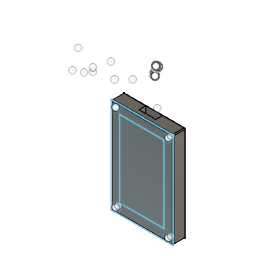
macropad-design 3.0 (Autodesk Fusion 360 design; units mm, degrees)
part number: 2025-12-03-17-34-09-700
part number: 2026-05-21-03-28-54-100
Autodesk Fusion 360 part; units mm, degrees
sketch "Sketch1" plane through (0, 0, 0) normal (0, 1, 0) x (1, 0, 0)
  line L0 (-41.1708, 57.3999) -> (7.4423, 57.3999)
  line L1 (7.4423, 57.3999) -> (7.4423, 141.552)
  line L2 (7.4423, 141.552) -> (-41.1708, 141.552)
  line L3 (-41.1708, 141.552) -> (-41.1708, 57.3999)
  line L4 (-50.6708, 47.8999) -> (17.375, 47.8999)
  line L5 (17.375, 47.8999) -> (17.375, 152.9579)
  line L6 (17.375, 152.9579) -> (-50.6708, 152.9579)
  line L7 (-50.6708, 152.9579) -> (-50.6708, 47.8999)
  circle A0 centre (-45.6708, 147.9579) radius 1.7
  circle A1 centre (-45.6708, 52.8999) radius 1.7
  circle A2 centre (12.375, 52.8999) radius 1.7
  circle A3 centre (12.375, 147.9579) radius 1.7
  circle A4 centre (-45.6708, 52.8999) radius 3
  circle A5 centre (12.375, 52.8999) radius 3
  circle A6 centre (12.375, 147.9579) radius 3
  circle A7 centre (-45.6708, 147.9579) radius 3
  dimension "d1" = 105.058
  dimension "d2" = 68.0458
  dimension "d3" = 48.6131
  dimension "d4" = 84.1522
  dimension "d5" = 9.5
  dimension "d6" = 9.5
  dimension "d7" = 3.4
  dimension "d8" = 5
  dimension "d9" = 5
  dimension "d10" = 3.4
  dimension "d11" = 5
  dimension "d12" = 5
  dimension "d13" = 3.4
  dimension "d14" = 5
  dimension "d15" = 5
  dimension "d16" = 3.4
  dimension "d17" = 5
  dimension "d18" = 5
  dimension "d19" = 6
  dimension "d20" = 6
  dimension "d21" = 6
  dimension "d22" = 6
  constraint horizontal L0
  constraint vertical L1
  constraint horizontal L2
  constraint vertical L3
  constraint horizontal L4
  constraint vertical L5
  constraint horizontal L6
  constraint vertical L7
  constraint concentric A1 A4
  constraint concentric A2 A5
  constraint concentric A3 A6
  constraint concentric A0 A7
  measures "d1" distance of L4.end L5.end
  measures "d2" distance of L4.start L4.end
  measures "d3" distance of L0.start L0.end
  measures "d4" distance of L0.start L2.end
  measures "d5" distance of L3 L7
  measures "d6" distance of L0 L4
  measures "d7" diameter of A0
  measures "d8" distance of L7 A0.centre
  measures "d9" distance of L6 A0.centre
  measures "d10" diameter of A1
  measures "d11" distance of L7 A1.centre
  measures "d12" distance of L4 A1.centre
  measures "d13" diameter of A2
  measures "d14" distance of L5 A2.centre
  measures "d15" distance of L4 A2.centre
  measures "d16" diameter of A3
  measures "d17" distance of L6 A3.centre
  measures "d18" distance of L5 A3.centre
  measures "d19" diameter of A4
  measures "d20" diameter of A5
  measures "d21" diameter of A6
  measures "d22" diameter of A7
extrude "Extrude1" add sketch "Sketch1" along normal blind 9.9 from surface at 3.1 contours A4 | A5 | A6 | A7 makes body 1 at (-48.667, 9.7, -52.7503) makes body 2 at (-42.9063, 9.7, -149.1232) makes body 3 at (15.3713, 9.7, -52.7503) makes body 4 at (9.6106, 9.7, -149.1232)
extrude "Extrude2" add sketch "Sketch1" along normal blind 13 contours L4 L5 L6 L7 bodies 1 2 3 4
extrude "Extrude3" add sketch "Sketch1" along normal blind 3 contours L0 L1 L2 L3 bodies 1
sketch "Sketch2" plane through (0, 13, 0) normal (0, 1, 0) x (-1, 0, 0)
  circle A0 centre (45.6708, -52.8999) radius 1.7
  circle A1 centre (-12.375, -147.9579) radius 1.7
  line L0 (41.1708, -57.3999) -> (41.1708, -141.552)
  line L1 (41.1708, -141.552) -> (-7.4423, -141.552)
  line L2 (-7.4423, -141.552) -> (-7.4423, -57.3999)
  line L3 (-7.4423, -57.3999) -> (41.1708, -57.3999)
  line L4 (50.6708, -152.9579) -> (50.6708, -47.8999)
  line L5 (50.6708, -47.8999) -> (-17.375, -47.8999)
  line L6 (-17.375, -47.8999) -> (-17.375, -152.9579)
  line L7 (-17.375, -152.9579) -> (50.6708, -152.9579)
  circle A2 centre (45.6708, -147.9579) radius 1.7
  circle A3 centre (-12.375, -52.8999) radius 1.7
  line L8 (7.175, -47.8999) -> (25.675, -47.8999)
  line L9 (25.675, -47.8999) -> (25.675, -57.3999)
  line L10 (25.675, -57.3999) -> (7.175, -57.3999)
  line L11 (7.175, -57.3999) -> (7.175, -47.8999)
  line L12 (-17.375, -47.8999) -> (-17.375, -152.9579)
  line L13 (-17.375, -152.9579) -> (50.6708, -152.9579)
  line L14 (50.6708, -152.9579) -> (50.6708, -47.8999)
  line L15 (50.6708, -47.8999) -> (-17.375, -47.8999)
  line L16 (-17.375, -47.8999) -> (-17.375, -152.9579)
  point P0 (50.6708, -152.9579)
  point P1 (-17.375, -152.9579)
  point P2 (50.6708, -47.8999)
  point P3 (-17.375, -47.8999)
  dimension "d30" = 18.5
  dimension "d32" = 24.55
  constraint horizontal L8
  constraint vertical L9
  constraint horizontal L10
  constraint vertical L11
  constraint coincident L5 L8.start
  measures "d30" distance of L8.start L8.end
  measures "d32" distance of L11 L12
extrude "Extrude4" cut sketch "Sketch2" against normal blind 7.5 contours L3 L5 L8 L9 L10 L11 L15 bodies 1
sketch "Sketch3" plane through (0, 0, 0) normal (0, 1, 0) x (1, 0, 0)
sketch "Sketch4" plane through (0, 3, 0) normal (0, 1, 0) x (-1, 0, 0)
  line L0 (41.1708, -141.552) -> (41.1708, -57.3999)
  line L1 (41.1708, -57.3999) -> (-7.4423, -57.3999)
  line L2 (-7.4423, -57.3999) -> (-7.4423, -141.552)
  line L3 (-7.4423, -141.552) -> (41.1708, -141.552)
  line L4 (6.8441, -1.7803) -> (6.8447, -1.7809)
  line L5 (6.8447, -1.7809) -> (6.8447, -1.7812)
  line L6 (6.8447, -1.7812) -> (6.8447, -5.0625)
  line L7 (6.8447, -5.0625) -> (6.8447, -5.0629)
  line L8 (6.8447, -5.0629) -> (6.8441, -5.0634)
  line L9 (6.8441, -5.0634) -> (6.8438, -5.0635)
  line L10 (6.8438, -5.0635) -> (4.9688, -5.0635)
  line L11 (4.9688, -5.0635) -> (4.9684, -5.0634)
  line L12 (4.9684, -5.0634) -> (4.9678, -5.0629)
  line L13 (4.9678, -5.0629) -> (4.9678, -5.0625)
  line L14 (4.9678, -5.0625) -> (4.9678, -1.7812)
  line L15 (4.9678, -1.7812) -> (4.9678, -1.7809)
  line L16 (4.9678, -1.7809) -> (4.9684, -1.7803)
  line L17 (4.9684, -1.7803) -> (4.9688, -1.7803)
  line L18 (4.9688, -1.7803) -> (6.8438, -1.7803)
  line L19 (6.8438, -1.7803) -> (6.8441, -1.7803)
  line L20 (4.9697, -1.7822) -> (4.9697, -5.0615)
  line L21 (4.9697, -5.0615) -> (6.8428, -5.0615)
  line L22 (6.8428, -5.0615) -> (6.8428, -1.7822)
  line L23 (6.8428, -1.7822) -> (4.9697, -1.7822)
  circle A0 centre (6.75, -4.9688) radius 0.0433
  circle A1 centre (5.0625, -4.9688) radius 0.0433
  circle A2 centre (6.75, -1.875) radius 0.0433
  circle A3 centre (5.0625, -1.875) radius 0.0433
  circle A4 centre (5.3312, -3.0938) radius 0.0335
  circle A5 centre (5.5312, -3.0938) radius 0.0787
  circle A6 centre (5.7313, -3.0938) radius 0.0335
  circle A7 centre (5.6312, -2.8937) radius 0.0295
  circle A8 centre (5.3812, -2.9937) radius 0.0295
  circle A9 centre (6.0813, -3.0938) radius 0.0335
  circle A10 centre (6.2812, -3.0938) radius 0.0787
  circle A11 centre (6.4813, -3.0938) radius 0.0335
  circle A12 centre (6.3813, -2.8937) radius 0.0295
  circle A13 centre (6.1313, -2.9937) radius 0.0295
  circle A14 centre (5.5858, -1.8956) radius 0.0175
  circle A15 centre (5.5858, -1.9956) radius 0.0175
  circle A16 centre (5.5858, -2.0956) radius 0.0175
  circle A17 centre (5.5858, -2.1956) radius 0.0175
  circle A18 centre (5.5858, -2.2956) radius 0.0175
  circle A19 centre (5.5858, -2.3956) radius 0.0175
  circle A20 centre (5.5858, -2.4956) radius 0.0175
  circle A21 centre (6.1858, -2.4956) radius 0.0175
  circle A22 centre (6.1858, -2.3956) radius 0.0175
  circle A23 centre (6.1858, -2.2956) radius 0.0175
  circle A24 centre (6.1858, -2.1956) radius 0.0175
  circle A25 centre (6.1858, -2.0956) radius 0.0175
  circle A26 centre (6.1858, -1.9956) radius 0.0175
  circle A27 centre (6.1858, -1.8956) radius 0.0175
  circle A28 centre (6.0813, -3.8438) radius 0.0335
  circle A29 centre (6.2812, -3.8438) radius 0.0787
  circle A30 centre (6.4813, -3.8438) radius 0.0335
  circle A31 centre (6.3813, -3.6437) radius 0.0295
  circle A32 centre (6.1313, -3.7438) radius 0.0295
  circle A33 centre (5.3312, -3.8438) radius 0.0335
  circle A34 centre (5.5312, -3.8438) radius 0.0787
  circle A35 centre (5.7313, -3.8438) radius 0.0335
  circle A36 centre (5.6312, -3.6437) radius 0.0295
  circle A37 centre (5.3812, -3.7438) radius 0.0295
  circle A38 centre (5.3312, -4.5938) radius 0.0335
  circle A39 centre (5.5312, -4.5938) radius 0.0787
  circle A40 centre (5.7313, -4.5938) radius 0.0335
  circle A41 centre (5.6312, -4.3937) radius 0.0295
  circle A42 centre (5.3812, -4.4938) radius 0.0295
  circle A43 centre (6.75, -4.9688) radius 0.0433
  circle A44 centre (5.0625, -4.9688) radius 0.0433
  circle A45 centre (6.75, -1.875) radius 0.0433
  circle A46 centre (5.0625, -1.875) radius 0.0433
  circle A47 centre (5.3312, -3.0938) radius 0.0335
  circle A48 centre (5.5312, -3.0938) radius 0.0787
  circle A49 centre (5.7313, -3.0938) radius 0.0335
  circle A50 centre (5.6312, -2.8937) radius 0.0295
  circle A51 centre (5.3812, -2.9937) radius 0.0295
  circle A52 centre (6.0813, -3.0938) radius 0.0335
  circle A53 centre (6.2812, -3.0938) radius 0.0787
  circle A54 centre (6.4813, -3.0938) radius 0.0335
  circle A55 centre (6.3813, -2.8937) radius 0.0295
  circle A56 centre (6.1313, -2.9937) radius 0.0295
  circle A57 centre (5.5858, -1.8956) radius 0.0175
  circle A58 centre (5.5858, -1.9956) radius 0.0175
  circle A59 centre (5.5858, -2.0956) radius 0.0175
  circle A60 centre (5.5858, -2.1956) radius 0.0175
  circle A61 centre (5.5858, -2.2956) radius 0.0175
  circle A62 centre (5.5858, -2.3956) radius 0.0175
  circle A63 centre (5.5858, -2.4956) radius 0.0175
  circle A64 centre (6.1858, -2.4956) radius 0.0175
  circle A65 centre (6.1858, -2.3956) radius 0.0175
  circle A66 centre (6.1858, -2.2956) radius 0.0175
  circle A67 centre (6.1858, -2.1956) radius 0.0175
  circle A68 centre (6.1858, -2.0956) radius 0.0175
  circle A69 centre (6.1858, -1.9956) radius 0.0175
  circle A70 centre (6.1858, -1.8956) radius 0.0175
  circle A71 centre (6.0813, -3.8438) radius 0.0335
  circle A72 centre (6.2812, -3.8438) radius 0.0787
  circle A73 centre (6.4813, -3.8438) radius 0.0335
  circle A74 centre (6.3813, -3.6437) radius 0.0295
  circle A75 centre (6.1313, -3.7438) radius 0.0295
  circle A76 centre (5.3312, -3.8438) radius 0.0335
  circle A77 centre (5.5312, -3.8438) radius 0.0787
  circle A78 centre (5.7313, -3.8438) radius 0.0335
  circle A79 centre (5.6312, -3.6437) radius 0.0295
  circle A80 centre (5.3812, -3.7438) radius 0.0295
  circle A81 centre (5.3312, -4.5938) radius 0.0335
  circle A82 centre (5.5312, -4.5938) radius 0.0787
  circle A83 centre (5.7313, -4.5938) radius 0.0335
  circle A84 centre (5.6312, -4.3937) radius 0.0295
  circle A85 centre (5.3812, -4.4938) radius 0.0295
  circle A86 centre (45.6105, -147.9399) radius 2.5
  circle A87 centre (-12.2673, -147.927) radius 2.5
  circle A88 through (48.1716, -52.8994, -3) (44.4216, -50.7343, -3) (44.4216, -55.0645, -3)
  circle A89 centre (-12.3196, -52.8556) radius 2.5
  dimension "d35" = 5
  dimension "d36" = 5
  dimension "d37" = 5
  dimension "d38" = 5
  measures "d35" diameter of A86
  measures "d36" diameter of A87
  measures "d38" diameter of A89
extrude "Extrude5" cut sketch "Sketch4" along normal blind 6.4 contours A86 bodies 1
sketch "macropad-Edge_Cuts" plane through (0, 3, 0) normal (0, 1, 0) x (0, 0, 1)
  line L0 (6.8441, -1.7803) -> (6.8447, -1.7809)
  line L1 (6.8447, -1.7809) -> (6.8447, -1.7812)
  line L2 (6.8447, -1.7812) -> (6.8447, -5.0625)
  line L3 (6.8447, -5.0625) -> (6.8447, -5.0629)
  line L4 (6.8447, -5.0629) -> (6.8441, -5.0634)
  line L5 (6.8441, -5.0634) -> (6.8438, -5.0635)
  line L6 (6.8438, -5.0635) -> (4.9688, -5.0635)
  line L7 (4.9688, -5.0635) -> (4.9684, -5.0634)
  line L8 (4.9684, -5.0634) -> (4.9678, -5.0629)
  line L9 (4.9678, -5.0629) -> (4.9678, -5.0625)
  line L10 (4.9678, -5.0625) -> (4.9678, -1.7812)
  line L11 (4.9678, -1.7812) -> (4.9678, -1.7809)
  line L12 (4.9678, -1.7809) -> (4.9684, -1.7803)
  line L13 (4.9684, -1.7803) -> (4.9688, -1.7803)
  line L14 (4.9688, -1.7803) -> (6.8438, -1.7803)
  line L15 (6.8438, -1.7803) -> (6.8441, -1.7803)
  line L16 (4.9697, -1.7822) -> (4.9697, -5.0615)
  line L17 (4.9697, -5.0615) -> (6.8428, -5.0615)
  line L18 (6.8428, -5.0615) -> (6.8428, -1.7822)
  line L19 (6.8428, -1.7822) -> (4.9697, -1.7822)
  circle A0 centre (6.75, -4.9688) radius 0.0433
  circle A1 centre (-33.7206, -2.9937) radius 0.0433
  circle A2 centre (6.75, -1.875) radius 0.0433
  circle A3 centre (5.0625, -1.875) radius 0.0433
  circle A4 centre (5.3312, -3.0938) radius 0.0335
  circle A5 centre (5.5312, -3.0938) radius 0.0787
  circle A6 centre (5.7313, -3.0938) radius 0.0335
  circle A7 centre (5.6312, -2.8937) radius 0.0295
  circle A8 centre (5.3812, -2.9937) radius 0.0295
  circle A9 centre (6.0813, -3.0938) radius 0.0335
  circle A10 centre (6.2812, -3.0938) radius 0.0787
  circle A11 centre (6.4813, -3.0938) radius 0.0335
  circle A12 centre (6.3813, -2.8937) radius 0.0295
  circle A13 centre (6.1313, -2.9937) radius 0.0295
  circle A14 centre (5.5858, -1.8956) radius 0.0175
  circle A15 centre (5.5858, -1.9956) radius 0.0175
  circle A16 centre (5.5858, -2.0956) radius 0.0175
  circle A17 centre (5.5858, -2.1956) radius 0.0175
  circle A18 centre (5.5858, -2.2956) radius 0.0175
  circle A19 centre (5.5858, -2.3956) radius 0.0175
  circle A20 centre (5.5858, -2.4956) radius 0.0175
  circle A21 centre (6.1858, -2.4956) radius 0.0175
  circle A22 centre (6.1858, -2.3956) radius 0.0175
  circle A23 centre (6.1858, -2.2956) radius 0.0175
  circle A24 centre (6.1858, -2.1956) radius 0.0175
  circle A25 centre (6.1858, -2.0956) radius 0.0175
  circle A26 centre (6.1858, -1.9956) radius 0.0175
  circle A27 centre (6.1858, -1.8956) radius 0.0175
  circle A28 centre (6.0813, -3.8438) radius 0.0335
  circle A29 centre (6.2812, -3.8438) radius 0.0787
  circle A30 centre (6.4813, -3.8438) radius 0.0335
  circle A31 centre (6.3813, -3.6437) radius 0.0295
  circle A32 centre (6.1313, -3.7438) radius 0.0295
  circle A33 centre (5.3312, -3.8438) radius 0.0335
  circle A34 centre (5.5312, -3.8438) radius 0.0787
  circle A35 centre (5.7313, -3.8438) radius 0.0335
  circle A36 centre (5.6312, -3.6437) radius 0.0295
  circle A37 centre (-20, -90) radius 0.0295
  circle A38 centre (5.3312, -4.5938) radius 0.0335
  circle A39 centre (5.5312, -4.5938) radius 0.0787
  circle A40 centre (-20, -30) radius 0.0335
  circle A41 centre (5.6312, -4.3937) radius 0.0295
  circle A42 centre (5.3812, -4.4938) radius 0.0295
  circle A43 centre (-34.7247, -73.7928) radius 0.0433
  circle A44 centre (5.0625, -4.9688) radius 0.0433
  circle A45 centre (6.75, -1.875) radius 0.0433
  circle A46 centre (5.0625, -1.875) radius 0.0433
  circle A47 centre (5.3312, -3.0938) radius 0.0335
  circle A48 centre (5.5312, -3.0938) radius 0.0787
  circle A49 centre (5.7313, -3.0938) radius 0.0335
  circle A50 centre (5.6312, -2.8937) radius 0.0295
  circle A51 centre (5.3812, -2.9937) radius 0.0295
  circle A52 centre (6.0813, -3.0938) radius 0.0335
  circle A53 centre (6.2812, -3.0938) radius 0.0787
  circle A54 centre (6.4813, -3.0938) radius 0.0335
  circle A55 centre (6.3813, -2.8937) radius 0.0295
  circle A56 centre (6.1313, -2.9937) radius 0.0295
  circle A57 centre (5.5858, -1.8956) radius 0.0175
  circle A58 centre (5.5858, -1.9956) radius 0.0175
  circle A59 centre (5.5858, -2.0956) radius 0.0175
  circle A60 centre (5.5858, -2.1956) radius 0.0175
  circle A61 centre (5.5858, -2.2956) radius 0.0175
  circle A62 centre (5.5858, -2.3956) radius 0.0175
  circle A63 centre (5.5858, -2.4956) radius 0.0175
  circle A64 centre (6.1858, -2.4956) radius 0.0175
  circle A65 centre (6.1858, -2.3956) radius 0.0175
  circle A66 centre (6.1858, -2.2956) radius 0.0175
  circle A67 centre (6.1858, -2.1956) radius 0.0175
  circle A68 centre (6.1858, -2.0956) radius 0.0175
  circle A69 centre (6.1858, -1.9956) radius 0.0175
  circle A70 centre (6.1858, -1.8956) radius 0.0175
  circle A71 centre (-40.0793, -83.4982) radius 0.0335
  circle A72 centre (6.2812, -3.8438) radius 0.0787
  circle A73 centre (6.4813, -3.8438) radius 0.0335
  circle A74 centre (6.3813, -3.6437) radius 0.0295
  circle A75 centre (-30.374, -73.7928) radius 0.0295
  circle A76 centre (-30, -50) radius 0.0335
  circle A77 centre (5.5312, -3.8438) radius 0.0787
  circle A78 centre (5.7313, -3.8438) radius 0.0335
  circle A79 centre (5.6312, -3.6437) radius 0.0295
  circle A80 centre (-14.9792, -54.0474) radius 0.0295
  circle A81 centre (5.3312, -4.5938) radius 0.0335
  circle A82 centre (5.5312, -4.5938) radius 0.0787
  circle A83 centre (5.7313, -4.5938) radius 0.0335
  circle A84 centre (-44.43, -96.2155) radius 0.0295
  circle A85 centre (5.3812, -4.4938) radius 0.0295
extrude "Extrude6" add sketch "Sketch2" along normal blind 1.5 separate body makes body 5
sketch "Sketch6" plane through (0, 14.5, 0) normal (0, 1, 0) x (-1, 0, 0)
  circle A0 centre (45.6708, -147.9579) radius 1.7
  circle A1 centre (-12.375, -147.9579) radius 1.7
  circle A2 centre (45.6708, -52.8999) radius 1.7
  circle A3 centre (-12.375, -52.8999) radius 1.7
  line L0 (-17.375, -47.8999) -> (-17.375, -152.9579)
  line L1 (-17.375, -152.9579) -> (50.6708, -152.9579)
  line L2 (50.6708, -152.9579) -> (50.6708, -47.8999)
  line L3 (50.6708, -47.8999) -> (-17.375, -47.8999)
  line L4 (-7.3078, -140.6749) -> (-7.3213, -140.6614)
  line L5 (-7.3213, -140.6614) -> (-7.3232, -140.6519)
  line L6 (-7.3232, -140.6519) -> (-7.3232, -57.5509)
  line L7 (-7.3232, -57.5509) -> (-7.3213, -57.5414)
  line L8 (-7.3213, -57.5414) -> (-7.3078, -57.5279)
  line L9 (-7.3078, -57.5279) -> (-7.2983, -57.526)
  line L10 (-7.2983, -57.526) -> (40.188, -57.526)
  line L11 (40.188, -57.526) -> (40.1975, -57.5279)
  line L12 (40.1975, -57.5279) -> (40.211, -57.5414)
  line L13 (40.211, -57.5414) -> (40.2129, -57.5509)
  line L14 (40.2129, -57.5509) -> (40.2129, -140.6519)
  line L15 (40.2129, -140.6519) -> (40.211, -140.6614)
  line L16 (40.211, -140.6614) -> (40.1975, -140.6749)
  line L17 (40.1975, -140.6749) -> (40.188, -140.6768)
  line L18 (40.188, -140.6768) -> (-7.2983, -140.6768)
  line L19 (-7.2983, -140.6768) -> (-7.3078, -140.6749)
  line L20 (40.163, -140.6269) -> (40.163, -57.5758)
  line L21 (40.163, -57.5758) -> (-7.2734, -57.5758)
  line L22 (-7.2734, -57.5758) -> (-7.2734, -140.6269)
  line L23 (-7.2734, -140.6269) -> (40.163, -140.6269)
  circle A4 centre (-4.924, -59.9252) radius 1.0968
  circle A5 centre (37.8137, -59.9252) radius 1.0968
  circle A6 centre (-4.924, -138.2775) radius 1.0968
  circle A7 centre (37.8137, -138.2775) radius 1.0968
  circle A8 centre (31.0073, -107.4115) radius 0.8475
  circle A9 centre (25.9421, -107.4115) radius 1.9942
  circle A10 centre (20.8769, -107.4115) radius 0.8475
  circle A11 centre (23.4095, -112.4767) radius 0.7478
  circle A12 centre (29.741, -109.9441) radius 0.7478
  circle A13 centre (12.0128, -107.4115) radius 0.8475
  circle A14 centre (6.9476, -107.4115) radius 1.9942
  circle A15 centre (1.8824, -107.4115) radius 0.8475
  circle A16 centre (4.415, -112.4767) radius 0.7478
  circle A17 centre (10.7465, -109.9441) radius 0.7478
  circle A18 centre (24.5599, -137.7556) radius 0.4432
  circle A19 centre (24.5599, -135.223) radius 0.4432
  circle A20 centre (24.5599, -132.6904) radius 0.4432
  circle A21 centre (24.5599, -130.1578) radius 0.4432
  circle A22 centre (24.5599, -127.6252) radius 0.4432
  circle A23 centre (24.5599, -125.0926) radius 0.4432
  circle A24 centre (24.5599, -122.56) radius 0.4432
  circle A25 centre (9.3643, -122.56) radius 0.4432
  circle A26 centre (9.3643, -125.0926) radius 0.4432
  circle A27 centre (9.3643, -127.6252) radius 0.4432
  circle A28 centre (9.3643, -130.1578) radius 0.4432
  circle A29 centre (9.3643, -132.6904) radius 0.4432
  circle A30 centre (9.3643, -135.223) radius 0.4432
  circle A31 centre (9.3643, -137.7556) radius 0.4432
  circle A32 centre (12.0128, -88.417) radius 0.8475
  circle A33 centre (6.9476, -88.417) radius 1.9942
  circle A34 centre (1.8824, -88.417) radius 0.8475
  circle A35 centre (4.415, -93.4822) radius 0.7478
  circle A36 centre (10.7465, -90.9496) radius 0.7478
  circle A37 centre (31.0073, -88.417) radius 0.8475
  circle A38 centre (25.9421, -88.417) radius 1.9942
  circle A39 centre (20.8769, -88.417) radius 0.8475
  circle A40 centre (23.4095, -93.4822) radius 0.7478
  circle A41 centre (29.741, -90.9496) radius 0.7478
  circle A42 centre (31.0073, -69.4225) radius 0.8475
  circle A43 centre (25.9421, -69.4225) radius 1.9942
  circle A44 centre (20.8769, -69.4225) radius 0.8475
  circle A45 centre (23.4095, -74.4877) radius 0.7478
  circle A46 centre (29.741, -71.9551) radius 0.7478
  circle A47 centre (-4.924, -59.9252) radius 1.0968
  circle A48 centre (37.8137, -59.9252) radius 1.0968
  circle A49 centre (-4.924, -138.2775) radius 1.0968
  circle A50 centre (37.8137, -138.2775) radius 1.0968
  circle A51 centre (31.0073, -107.4115) radius 0.8475
  circle A52 centre (25.9421, -107.4115) radius 1.9942
  circle A53 centre (20.8769, -107.4115) radius 0.8475
  circle A54 centre (23.4095, -112.4767) radius 0.7478
  circle A55 centre (29.741, -109.9441) radius 0.7478
  circle A56 centre (12.0128, -107.4115) radius 0.8475
  circle A57 centre (6.9476, -107.4115) radius 1.9942
  circle A58 centre (1.8824, -107.4115) radius 0.8475
  circle A59 centre (4.415, -112.4767) radius 0.7478
  circle A60 centre (10.7465, -109.9441) radius 0.7478
  circle A61 centre (24.5599, -137.7556) radius 0.4432
  circle A62 centre (24.5599, -135.223) radius 0.4432
  circle A63 centre (24.5599, -132.6904) radius 0.4432
  circle A64 centre (24.5599, -130.1578) radius 0.4432
  circle A65 centre (24.5599, -127.6252) radius 0.4432
  circle A66 centre (24.5599, -125.0926) radius 0.4432
  circle A67 centre (24.5599, -122.56) radius 0.4432
  circle A68 centre (9.3643, -122.56) radius 0.4432
  circle A69 centre (9.3643, -125.0926) radius 0.4432
  circle A70 centre (9.3643, -127.6252) radius 0.4432
  circle A71 centre (9.3643, -130.1578) radius 0.4432
  circle A72 centre (9.3643, -132.6904) radius 0.4432
  circle A73 centre (9.3643, -135.223) radius 0.4432
  circle A74 centre (9.3643, -137.7556) radius 0.4432
  circle A75 centre (12.0128, -88.417) radius 0.8475
  circle A76 centre (6.9476, -88.417) radius 1.9942
  circle A77 centre (1.8824, -88.417) radius 0.8475
  circle A78 centre (4.415, -93.4822) radius 0.7478
  circle A79 centre (10.7465, -90.9496) radius 0.7478
  circle A80 centre (31.0073, -88.417) radius 0.8475
  circle A81 centre (25.9421, -88.417) radius 1.9942
  circle A82 centre (20.8769, -88.417) radius 0.8475
  circle A83 centre (23.4095, -93.4822) radius 0.7478
  circle A84 centre (29.741, -90.9496) radius 0.7478
  circle A85 centre (31.0073, -69.4225) radius 0.8475
  circle A86 centre (25.9421, -69.4225) radius 1.9942
  circle A87 centre (20.8769, -69.4225) radius 0.8475
  circle A88 centre (23.4095, -74.4877) radius 0.7478
  circle A89 centre (29.741, -71.9551) radius 0.7478
  line L24 (0.9476, -82.417) -> (12.9476, -82.417)
  line L25 (12.9476, -82.417) -> (12.9476, -94.417)
  line L26 (12.9476, -94.417) -> (0.9476, -94.417)
  line L27 (0.9476, -94.417) -> (0.9476, -82.417)
  line L28 (0.9476, -82.417) -> (12.9476, -94.417) construction
  line L29 (12.9476, -82.417) -> (0.9476, -94.417) construction
  line L30 (31.9421, -63.4225) -> (19.9421, -63.4225)
  line L31 (19.9421, -63.4225) -> (19.9421, -75.4225)
  line L32 (19.9421, -75.4225) -> (31.9421, -75.4225)
  line L33 (31.9421, -75.4225) -> (31.9421, -63.4225)
  line L34 (31.9421, -63.4225) -> (19.9421, -75.4225) construction
  line L35 (19.9421, -63.4225) -> (31.9421, -75.4225) construction
  line L36 (31.9421, -82.417) -> (19.9421, -82.417)
  line L37 (19.9421, -82.417) -> (19.9421, -94.417)
  line L38 (19.9421, -94.417) -> (31.9421, -94.417)
  line L39 (31.9421, -94.417) -> (31.9421, -82.417)
  line L40 (31.9421, -82.417) -> (19.9421, -94.417) construction
  line L41 (19.9421, -82.417) -> (31.9421, -94.417) construction
  line L42 (12.9476, -101.4115) -> (0.9476, -101.4115)
  line L43 (0.9476, -101.4115) -> (0.9476, -113.4115)
  line L44 (0.9476, -113.4115) -> (12.9476, -113.4115)
  line L45 (12.9476, -113.4115) -> (12.9476, -101.4115)
  line L46 (12.9476, -101.4115) -> (0.9476, -113.4115) construction
  line L47 (0.9476, -101.4115) -> (12.9476, -113.4115) construction
  line L48 (19.9421, -101.4115) -> (31.9421, -101.4115)
  line L49 (31.9421, -101.4115) -> (31.9421, -113.4115)
  line L50 (31.9421, -113.4115) -> (19.9421, -113.4115)
  line L51 (19.9421, -113.4115) -> (19.9421, -101.4115)
  line L52 (19.9421, -101.4115) -> (31.9421, -113.4115) construction
  line L53 (31.9421, -101.4115) -> (19.9421, -113.4115) construction
  line L54 (13.9476, -81.417) -> (-0.0524, -81.417)
  line L55 (-0.0524, -81.417) -> (-0.0524, -95.417)
  line L56 (-0.0524, -95.417) -> (13.9476, -95.417)
  line L57 (13.9476, -95.417) -> (13.9476, -81.417)
  line L58 (13.9476, -81.417) -> (-0.0524, -95.417) construction
  line L59 (-0.0524, -81.417) -> (13.9476, -95.417) construction
  line L60 (18.9421, -62.4225) -> (32.9421, -62.4225)
  line L61 (32.9421, -62.4225) -> (32.9421, -76.4225)
  line L62 (32.9421, -76.4225) -> (18.9421, -76.4225)
  line L63 (18.9421, -76.4225) -> (18.9421, -62.4225)
  line L64 (18.9421, -62.4225) -> (32.9421, -76.4225) construction
  line L65 (32.9421, -62.4225) -> (18.9421, -76.4225) construction
  line L66 (18.9421, -81.417) -> (32.9421, -81.417)
  line L67 (32.9421, -81.417) -> (32.9421, -95.417)
  line L68 (32.9421, -95.417) -> (18.9421, -95.417)
  line L69 (18.9421, -95.417) -> (18.9421, -81.417)
  line L70 (18.9421, -81.417) -> (32.9421, -95.417) construction
  line L71 (32.9421, -81.417) -> (18.9421, -95.417) construction
  line L72 (-0.0524, -100.4115) -> (13.9476, -100.4115)
  line L73 (13.9476, -100.4115) -> (13.9476, -114.4115)
  line L74 (13.9476, -114.4115) -> (-0.0524, -114.4115)
  line L75 (-0.0524, -114.4115) -> (-0.0524, -100.4115)
  line L76 (-0.0524, -100.4115) -> (13.9476, -114.4115) construction
  line L77 (13.9476, -100.4115) -> (-0.0524, -114.4115) construction
  line L78 (18.9421, -100.4115) -> (32.9421, -100.4115)
  line L79 (32.9421, -100.4115) -> (32.9421, -114.4115)
  line L80 (32.9421, -114.4115) -> (18.9421, -114.4115)
  line L81 (18.9421, -114.4115) -> (18.9421, -100.4115)
  line L82 (18.9421, -100.4115) -> (32.9421, -114.4115) construction
  line L83 (32.9421, -100.4115) -> (18.9421, -114.4115) construction
  point P0 (6.9476, -88.417)
  point P1 (25.9421, -69.4225)
  point P2 (25.9421, -88.417)
  point P3 (6.9476, -107.4115)
  point P4 (25.9421, -107.4115)
  point P5 (6.9476, -88.417)
  point P6 (25.9421, -69.4225)
  point P7 (25.9421, -88.417)
  point P8 (6.9476, -107.4115)
  point P9 (25.9421, -107.4115)
  dimension "d43" = 12
  dimension "d44" = 12
  dimension "d45" = 12
  dimension "d46" = 12
  dimension "d47" = 12
  dimension "d48" = 12
  dimension "d49" = 12
  dimension "d50" = 12
  dimension "d51" = 12
  dimension "d52" = 12
  dimension "d57" = 14
  dimension "d58" = 14
  dimension "d59" = 14
  dimension "d60" = 14
  dimension "d61" = 14
  dimension "d62" = 14
  dimension "d63" = 14
  dimension "d64" = 14
  dimension "d65" = 14
  dimension "d66" = 14
  constraint horizontal L24
  constraint perpendicular L24 L25
  constraint parallel L24 L26
  constraint parallel L25 L27
  constraint coincident L28 P5
  constraint coincident L29 P5
  constraint coincident P5 P0
  constraint horizontal L30
  constraint perpendicular L30 L31
  constraint parallel L30 L32
  constraint parallel L31 L33
  constraint coincident L34 P6
  constraint coincident L35 P6
  constraint coincident P6 P1
  constraint horizontal L36
  constraint perpendicular L36 L37
  constraint parallel L36 L38
  constraint parallel L37 L39
  constraint coincident L40 P7
  constraint coincident L41 P7
  constraint coincident P7 P2
  constraint horizontal L42
  constraint perpendicular L42 L43
  constraint parallel L42 L44
  constraint parallel L43 L45
  constraint coincident L46 P8
  constraint coincident L47 P8
  constraint coincident P8 P3
  constraint horizontal L48
  constraint perpendicular L48 L49
  constraint parallel L48 L50
  constraint parallel L49 L51
  constraint coincident L52 P9
  constraint coincident L53 P9
  constraint coincident P9 P4
  constraint horizontal L54
  constraint perpendicular L54 L55
  constraint parallel L54 L56
  constraint parallel L55 L57
  constraint coincident L58 P5
  constraint coincident L59 P5
  constraint horizontal L60
  constraint perpendicular L60 L61
  constraint parallel L60 L62
  constraint parallel L61 L63
  constraint coincident L64 P6
  constraint coincident L65 P6
  constraint horizontal L66
  constraint perpendicular L66 L67
  constraint parallel L66 L68
  constraint parallel L67 L69
  constraint coincident L70 P7
  constraint coincident L71 P7
  constraint horizontal L72
  constraint perpendicular L72 L73
  constraint parallel L72 L74
  constraint parallel L73 L75
  constraint coincident L76 P8
  constraint coincident L77 P8
  constraint horizontal L78
  constraint perpendicular L78 L79
  constraint parallel L78 L80
  constraint parallel L79 L81
  constraint coincident L82 P9
  constraint coincident L83 P9
  measures "d43" distance of L25.end L26.end
  measures "d44" distance of L24.end L25.end
  measures "d45" distance of L31.end L32.end
  measures "d46" distance of L30.end L31.end
  measures "d47" distance of L37.end L38.end
  measures "d48" distance of L36.end L37.end
  measures "d49" distance of L43.end L44.end
  measures "d50" distance of L42.end L43.end
  measures "d51" distance of L49.end L50.end
  measures "d52" distance of L48.end L49.end
  measures "d57" distance of L55.end L56.end
  measures "d58" distance of L54.end L55.end
  measures "d59" distance of L61.end L62.end
  measures "d60" distance of L60.end L61.end
  measures "d61" distance of L67.end L68.end
  measures "d62" distance of L66.end L67.end
  measures "d63" distance of L73.end L74.end
  measures "d64" distance of L72.end L73.end
  measures "d65" distance of L79.end L80.end
  measures "d66" distance of L78.end L79.end
extrude "Extrude7" cut sketch "Sketch6" against normal blind 1.5 contours A8 A51 | A9 A52 | A10 A53 | A11 A54 | A12 A55 | A13 A56 | A14 A57 | A15 A58 | A16 A59 | A17 A60 | A32 A75 | A33 A76 | A34 A77 | A35 A78 | A36 A79 | A37 A80 | A38 A81 | A39 A82 | A40 A83 | A41 A84 | A42 A85 | A43 A86 | A44 A87 | A45 A88 | A46 A89 | L24 L25 L26 L27 | L30 L31 L32 L33 | L36 L37 L38 L39 | L42 L43 L44 L45 | L48 L49 L50 L51 bodies 5
fillet "Fillet1" radius 1 8 edges at (-50.6708, 6.5, -47.8999) (17.375, 6.5, -47.8999) (-16.6479, 0, -47.8999) (-50.6708, 0, -100.4289) (-50.6708, 6.5, -152.9579) (17.375, 0, -100.4289) (17.375, 6.5, -152.9579) (-16.6479, 0, -152.9579) on bodies 1
extrude "Extrude8" cut sketch "Sketch6" against normal blind 1.5 contours L24 L25 L26 L27 | L54 L55 L56 L57 bodies 5
extrude "Extrude9" cut sketch "Sketch6" against normal blind 1.5 contours L30 L31 L32 L33 | L36 L37 L38 L39 | L42 L43 L44 L45 | L48 L49 L50 L51 | L60 L61 L62 L63 | L66 L67 L68 L69 | L72 L73 L74 L75 | L78 L79 L80 L81 bodies 5
fillet "Fillet2" radius 1 2 edges at (-50.6708, 14.5, -100.4289) (-16.6479, 14.5, -152.9579) 1 faces at (-17.4126, 14.5, -136.6068) on bodies 5
component "top cover" placed x (1, 0, 0) y (0, 1, 0) z (0, 0, 1) at (0, 0, 0)
